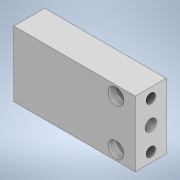
# Autodesk Inventor part: シリンダー
Saved by Autodesk Inventor 2022 (Build 260153070, 153G)
## iProperties
Created: 2022-09-26
Part Number: シリンダー
Material: 一般
Document SubType Name: Modeling
Designer: hirok
Density: 1 g/cm^3
Appearance: 既定
Author: hirok
Autodesk Inventor part; units mm, degrees
ref_plane "YZ Plane" through (0, 0, 0) normal (1, 0, 0) x (0, 1, 0)
ref_plane "XZ Plane" through (0, 0, 0) normal (0, 1, 0) x (-1, 0, 0)
ref_plane "XY Plane" through (0, 0, 0) normal (0, 0, 1) x (1, 0, 0)
sketch "スケッチ1" plane through (0, 0, 0) normal (0, 0, 1) x (1, 0, 0)
  line L0 (0, 0) -> (31.5, 0)
  line L1 (31.5, 0) -> (31.5, 17)
  line L2 (31.5, 17) -> (0, 17)
  line L3 (0, 17) -> (0, 0)
  dimension "d0" = 31.5
  dimension "d1" = 17
  constraints: 8 end point, 2 parallel, 1 horizontal, 1 perpendicular
  measures "d0" distance of L1.end L2.end
  measures "d1" distance of L2.end L0.start
extrude "押し出し1" add sketch "スケッチ1" along normal blind 8
sketch "スケッチ2" plane through (31.5, 0, 0) normal (1, 0, 0) x (0, 0, -1)
  line L0 (0, 17) -> (-8, 17) projected
  line L1 (0, 0) -> (0, 17) projected
  point P0 (-4, 8.5)
  dimension "d4" = 8.5
  dimension "d5" = 4
  measures "d4" distance from line of point (-4, 8.5) L0
  measures "d5" distance from line of L1 point (-4, 8.5)
hole "穴1" at (31.5, 8.5, 4) direction (-1, 0, 0) diameter 3 depth 20 tip angle 118
sketch "スケッチ3" plane through (31.5, 0, 0) normal (1, 0, 0) x (0, 0, -1)
  line L0 (-8, 0) -> (-8, 17) projected
  line L1 (-8, 8.5) -> (0, 8.5)
  line L2 (0, 0) -> (0, 17) projected
  line L3 (0, 17) -> (-8, 17) projected
  point P0 (-4, 14.5)
  point P1 (-4, 2.5)
  dimension "d13" = 2.5
  constraints: 2 end point, 2 midpoint, 1 symmetric about line
  measures "d13" distance from line of L3 point (-4, 14.5)
hole "穴2" at (31.5, 14.5, 4) at (31.5, 2.5, 4) direction (-1, 0, 0) diameter 2.459 depth 8.8 tip angle 118 thread size "M3x0.5" class "6H" standard "ISO Metric profile"
sketch "スケッチ4" plane through (0, 0, 8) normal (0, 0, 1) x (1, 0, 0)
  line L0 (31.5, 0) -> (31.5, 17) projected
  line L1 (31.5, 17) -> (0, 17) projected
  line L2 (0, 17) -> (0, 0) projected
  line L3 (0, 8.5) -> (31.5, 8.5)
  point P0 (26.5, 14.5)
  point P1 (26.5, 2.5)
  dimension "d21" = 5
  dimension "d22" = 2.5
  constraints: 2 end point, 2 midpoint, 1 symmetric about line
  measures "d21" distance from line of L0 point (26.5, 14.5)
  measures "d22" distance from line of L1 point (26.5, 14.5)
hole "穴3" at (26.5, 14.5, 8) at (26.5, 2.5, 8) direction (0, 0, -1) diameter 2.2 end through all
hole "穴4" at (26.5, 14.5, 8) at (26.5, 2.5, 8) direction (0, 0, -1) diameter 4.1 depth 2.2 tip angle 118
sketch "スケッチ5" plane through (0, 0, 0) normal (0, 0, -1) x (-1, 0, 0)
  line L0 (0, 0) -> (-31.5, 0) projected
  line L1 (-31.5, 0) -> (-31.5, 17) projected
  line L2 (0, 17) -> (0, 0) projected
  line L3 (0, 8.5) -> (-31.5, 8.5)
  line L4 (-31.5, 7) -> (-31.5, 10) projected
  point P0 (-26.5, 2.5)
  point P1 (-26.5, 14.5)
  dimension "d37" = 2.5
  dimension "d38" = 5
  constraints: 2 end point, 2 midpoint, 1 symmetric about line
  measures "d37" distance from line of L0 point (-26.5, 2.5)
  measures "d38" distance from line of L1 point (-26.5, 2.5)
hole "穴5" at (26.5, 2.5, 0) at (26.5, 14.5, 0) direction (0, 0, 1) diameter 4.1 depth 2.2 tip angle 118
sketch "スケッチ6" plane through (0, 0, 0) normal (0, -1, 0) x (1, 0, 0)
  line L0 (31.5, 0) -> (31.5, 8) projected
  point P0 (0, 0)
  point P1 (3, 4)
  point P2 (21.5, 4)
  dimension "d46" = 10
  dimension "d47" = 18.5
  measures "d46" distance from line of L0 point (21.5, 4)
  measures "d47" distance of point (21.5, 4) point (3, 4)
hole "穴6" at (3, 0, 4) at (21.5, 0, 4) direction (0, 1, 0) diameter 2.459 depth 8.8 tip angle 118 thread size "M3x0.5" class "6H" standard "ISO Metric profile"
